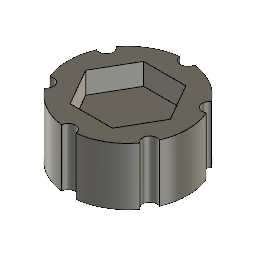
tapitaBase (Autodesk Fusion 360 design; units mm, degrees)
Autodesk Fusion 360 part; units mm, degrees
sketch "Boceto1" plane through (0, 0, 0) normal (0, 0, 1) x (1, 0, 0)
  line L0 (2.9445, -5.1) -> (5.889, 0)
  line L1 (5.889, 0) -> (2.9445, 5.1)
  line L2 (2.9445, 5.1) -> (-2.9445, 5.1)
  line L3 (-2.9445, 5.1) -> (-5.889, 0)
  line L4 (-5.889, 0) -> (-2.9445, -5.1)
  line L5 (-2.9445, -5.1) -> (2.9445, -5.1)
  circle A0 centre (0, 0) radius 8.3
  dimension "d1" = 5.1
  dimension "d2" = 16.6
  constraint coincident A0.centre origin
  measures "d1" distance of A0.centre L5
  measures "d2" diameter of A0
extrude "Extruir1" add sketch "Boceto1" along normal blind 8
extrude "Extruir2" add sketch "Boceto1" along normal blind 5 contours L0 L1 L2 L3 L4 L5
sketch "Boceto2" plane through (0, 0, 8) normal (0, 0, 1) x (-1, 0, 0)
  line L0 (-2.9445, 5.1) -> (2.9445, 5.1)
  line L1 (2.9445, 5.1) -> (5.889, 0)
  line L2 (5.889, 0) -> (2.9445, -5.1)
  line L3 (2.9445, -5.1) -> (-2.9445, -5.1)
  line L4 (-2.9445, -5.1) -> (-5.889, 0)
  line L5 (-5.889, 0) -> (-2.9445, 5.1)
  circle A0 centre (0, 0) radius 8.3
  circle A1 centre (0, -8.3) radius 1
  line L6 (0, 0) -> (0, -10.2342) construction
  circle A2 centre (7.188, -4.15) radius 1
  circle A3 centre (7.188, 4.15) radius 1
  circle A4 centre (0, 8.3) radius 1
  circle A5 centre (-7.188, 4.15) radius 1
  circle A6 centre (-7.188, -4.15) radius 1
  dimension "d7" = 2
  dimension "d9" = 360
  constraint coincident A0 A1.centre
  constraint coincident A0.centre L6.start
  constraint vertical L6
  constraint coincident A1.centre L6
  measures "d7" diameter of A1
extrude "Extruir3" cut sketch "Boceto2" against normal blind 8 contours A0 A3 | A0 A2 | A0 A4 | A0 A1 | A0 A5 | A0 A6 picked at (6.8842, 4.0023) picked at (6.8842, -4.0023) picked at (-0.024, 7.9631) picked at (-0.024, -7.9631) picked at (-6.9055, 3.9648) picked at (-6.9055, -3.9648)
